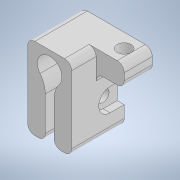
# Autodesk Inventor part: z belt clip
Saved by Autodesk Inventor 2022 (Build 260153000, 153)
## iProperties
Created: 2021-10-05
Part Number: z belt clip
Material: Generic
Document SubType Name: Modeling
Designer: Administrator
Density: 1 g/cm^3
Appearance: Default
Mass: 0.635636 g
Surface Area: 6.61381 cm^2
Volume: 0.635636 cm^3
Title: z belt clip v2
Author: Administrator
Autodesk Inventor part; units mm, degrees
ref_plane "YZ Plane" through (0, 0, 0) normal (1, 0, 0) x (0, 1, 0)
ref_plane "XZ Plane" through (0, 0, 0) normal (0, 1, 0) x (-1, 0, 0)
sketch "Sketch14" plane through (0, 0, 0) normal (0, 0, 1) x (1, 0, 0)
  circle A0 centre (0, 0) radius 3.5
  line L0 (-1.25, -3.2692) -> (1.25, -3.2692)
  line L1 (1.25, -3.2692) -> (1.25, -18.2692)
  line L2 (1.25, -18.2692) -> (-1.25, -18.2692)
  line L3 (-1.25, -18.2692) -> (-1.25, -3.2692)
  arc A1 (-1.25, -6.4952) -> (-2.75, -2.1651) centre (-8.25, -6.4952) ccw
  arc A2 (2.75, -2.1651) -> (1.25, -6.4952) centre (8.25, -6.4952) ccw
  line L4 (-6.25, 5) -> (6.25, 5)
  line L5 (6.25, 5) -> (6.25, -18.2692)
  line L6 (6.25, -18.2692) -> (-6.25, -18.2692)
  line L7 (-6.25, -18.2692) -> (-6.25, 5)
  point P0 (-1.25, -18.2692)
  point P1 (1.25, -18.2692)
  point P2 (-1.25, -18.2692)
  dimension "d67" = 7
  dimension "d68" = 2.5
  dimension "d69" = 7
  dimension "d70" = 7
  dimension "d71" = 15
  dimension "d72" = 5
  dimension "d73" = 5
  dimension "d74" = 5
  constraints: 16 end point, 8 point on circle, 4 parallel, 4 tangent, 3 centre point, 2 horizontal, 2 perpendicular, 2 point on line, 1 coincident, 1 collinear
  measures "d67" diameter of A0
  measures "d68" distance of L1.end L2.end
  measures "d69" radius of A2
  measures "d70" radius of A1
  measures "d71" distance of L0.end L1.end
  measures "d72" distance between parallel lines of L5 L1
  measures "d73" distance between parallel lines of L7 L3
  measures "d74" distance from line of L4 A0.centre
extrude "Extrusion8" add sketch "Sketch14" along normal blind 7 contours A0 A1 L3 L6 L7 L4 L5 L1 A2
extrude "Extrusion9" add sketch "Sketch14" against normal blind 8
hole "Hole12" at (0, 0, 0) direction (0, 0, -1) diameter 4 end through all
ref_plane "Work Plane4" through (-6.25, 2, 7) normal (0, 1, 0) x (1, 0, 0)
sketch "Sketch18" plane through (-6.25, 5, 7) normal (0, 1, 0) x (1, 0, 0)
  line L0 (12.5, 0) -> (12.5, 15) projected
  line L1 (12.5, 7) -> (20.5, 7)
  line L2 (20.5, 7) -> (20.5, 15)
  line L3 (20.5, 15) -> (12.5, 15)
  line L4 (12.5, 15) -> (12.5, 0)
  line L5 (0, 15) -> (12.5, 15) projected
  line L6 (20.5, 7) -> (12.5, 15) construction
  line L7 (19.25, 12.5877) -> (19.25, 9.4123)
  line L8 (19.25, 9.4123) -> (16.5, 7.8246)
  line L9 (16.5, 7.8246) -> (13.75, 9.4123)
  line L10 (13.75, 9.4123) -> (13.75, 12.5877)
  line L11 (13.75, 12.5877) -> (16.5, 14.1754)
  line L12 (16.5, 14.1754) -> (19.25, 12.5877)
  point P0 (6.25, 7)
  point P1 (16.5, 11)
  point P2 (16.5, 11)
  point P3 (12.5, 13)
  dimension "d112" = 8
  dimension "d113" = 5.5
  dimension "d139" = 8
  constraints: 22 end point, 2 parallel, 1 coincident, 1 collinear, 1 horizontal, 1 midpoint, 1 perpendicular, 1 point on line, 1 vertical, 13 other
  measures "d112" distance of L1.start L1.end
  measures "d113" distance between parallel lines of L7 L10
  measures "d139" distance of L1.end L2.end
extrude "Extrusion13" add sketch "Sketch18" against normal blind 6 contours L0 L3 L2 L1 | L7 L8 L9 L10 L11 L12
hole "Hole16" at (10.25, 5, -4) direction (0, -1, 0) diameter 4 end through all
sketch "Sketch19" plane through (6.25, -18.2692, 7) normal (1, 0, 0) x (0, 0, -1)
  line L0 (0, 0) -> (0, 11.774) projected
  line L1 (7, 0) -> (7, 11.774) projected
  line L2 (7, 11.774) -> (0, 11.774) projected
  line L3 (0, 0) -> (0, 11.774) projected
  line L4 (7, 0) -> (0, 0) projected
  line L5 (15, 17.2692) -> (7, 17.2692) projected
  line L6 (11, 8.6346) -> (11, 0) construction
  line L7 (7, 0) -> (15, 0) construction
  line L8 (15, 17.2692) -> (15, 0) construction
  line L9 (11, 8.6346) -> (11, 17.2692) construction
  point P0 (7, 18.2692)
  constraints: 6 end point, 2 midpoint, 2 vertical, 1 collinear, 1 horizontal
hole "Hole15" at (6.25, -9.6346, -4) direction (-1, 0, 0) diameter 3.4 end through all counterbore diameter 6.5 counterbore depth 2
sketch "Sketch20" plane through (6.25, -18.2692, 7) normal (1, 0, 0) x (0, 0, -1)
  line L0 (15, 17.2692) -> (15, 0) projected
  circle A0 centre (11, 8.6346) radius 3.25 projected
  circle A1 centre (11, 8.6346) radius 1.7 projected
  circle A2 centre (11, 8.6346) radius 3.25 projected
  line L1 (11, 5.3846) -> (11, 11.8846)
  line L2 (11, 11.8846) -> (15, 11.8846)
  line L3 (15, 11.8846) -> (15, 5.3846)
  line L4 (15, 5.3846) -> (11, 5.3846)
  point P0 (7, 18.2692)
  constraints: 8 end point, 2 parallel, 2 point on circle, 1 perpendicular, 1 vertical
extrude "Extrusion14" cut sketch "Sketch20" against normal up to surface (2 mm away) contours L0 L4 A0 L2 | A0 L1 A1 | A1 L1 picked at (13.692, 8.2674) picked at (11.6055, 9.0776)
fillet "Fillet3" radius 2 9 edges at (14.25, -1, -4) (-6.25, 5, -0.5) (-6.25, -18.2692, -0.5) (6.25, -18.2692, -0.5) (-1.25, -18.2692, 3.5) (1.25, -18.2692, 3.5) (6.25, -1, -4) (14.25, 5, -4) (6.25, 5, 3.5)
equation "\"d69\" = d67"
equation "\"d70\" = d67"
equation "\"d73\" = d72"
body "Solid6"
